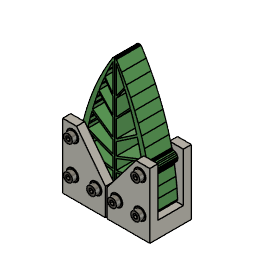
REVIEW_V2_ZeroGap_M3x30 (Autodesk Fusion 360 design; units mm, degrees)
part number: 2026-09-04-15-12-13-781
part number: 2026-09-04-15-12-27-275
part number: 2026-09-04-15-12-29-355
part number: 2026-09-04-15-12-34-345
part number: 2026-09-04-15-12-35-918
Autodesk Fusion 360 part; units mm, degrees
sketch "Single continuous Robotiq-to-UMI adapter envelope" plane through (0, 0, 0) normal (1, 0, 0) x (0, 0, -1) in component "LEFT V2 handed finger"
  line L0 (1, 0) -> (-25.7, 0)
  line L1 (-25.7, 0) -> (-25.7, 40.5)
  line L2 (-25.7, 40.5) -> (-17, 40.5)
  line L3 (-17, 40.5) -> (1, 17)
  line L4 (1, 17) -> (1, 0)
extrude "Extrude1" add sketch "Single continuous Robotiq-to-UMI adapter envelope" along normal mid plane 26 makes body 1 in component "LEFT V2 handed finger"
sketch "Continuous TPU pocket - 0.20 mm clearance per side" plane through (0, 0, 0) normal (0, 0, 1) x (1, 0, 0) in component "LEFT V2 handed finger"
  line L0 (-7.94, 10) -> (7.94, 10)
  line L1 (7.94, 10) -> (7.94, 100)
  line L2 (7.94, 100) -> (-7.94, 100)
  line L3 (-7.94, 100) -> (-7.94, 10)
extrude "Extrude2" cut sketch "Continuous TPU pocket - 0.20 mm clearance per side" along normal mid plane 100 bodies 1 in component "LEFT V2 handed finger"
sketch "Exact Robotiq M5 and indexing interface" plane through (0, 0, 0) normal (0, 1, 0) x (1, 0, 0) in component "LEFT V2 handed finger"
  circle A0 centre (0, -12.36) radius 2.65
  circle A1 centre (-4.5, -12.36) radius 1
  circle A2 centre (4.5, -12.36) radius 1
extrude "Extrude3" cut sketch "Exact Robotiq M5 and indexing interface" along normal blind 4 contours A0 bodies 1 in component "LEFT V2 handed finger"
extrude "Extrude4" cut sketch "Exact Robotiq M5 and indexing interface" along normal blind 2.5 contours A1 | A2 bodies 1 in component "LEFT V2 handed finger"
ref_plane "WorkPlane1" through (0, 4, 0) normal (0, 1, 0) x (0, 0, 1) in component "LEFT V2 handed finger"
sketch "Robotiq M5 SHCS head pocket - 9.2 mm" plane through (0, 4, 0) normal (0, 1, 0) x (1, 0, 0) in component "LEFT V2 handed finger"
  circle A0 centre (0, -12.36) radius 4.6
extrude "Extrude5" cut sketch "Robotiq M5 SHCS head pocket - 9.2 mm" along normal blind 6 bodies 1 in component "LEFT V2 handed finger"
sketch "Three UMI M3 holder clearances - 3.6 mm" plane through (0, 0, 0) normal (1, 0, 0) x (0, 0, -1) in component "LEFT V2 handed finger"
  circle A0 centre (-5, 13) radius 1.8
  circle A1 centre (-19.5, 13) radius 1.8
  circle A2 centre (-19.5, 34) radius 1.8
extrude "Extrude6" cut sketch "Three UMI M3 holder clearances - 3.6 mm" along normal mid plane 30 bodies 1 in component "LEFT V2 handed finger"
ref_plane "WorkPlane2" through (13, 0, 0) normal (1, 0, 0) x (0, 1, 0) in component "LEFT V2 handed finger"
sketch "Three shallow washer seats - 7.5 mm" plane through (13, 0, 0) normal (1, 0, 0) x (0, 0, -1) in component "LEFT V2 handed finger"
  circle A0 centre (-5, 13) radius 3.75
  circle A1 centre (-19.5, 13) radius 3.75
  circle A2 centre (-19.5, 34) radius 3.75
extrude "Extrude7" cut sketch "Three shallow washer seats - 7.5 mm" against normal blind 0.6 bodies 1 in component "LEFT V2 handed finger"
ref_plane "WorkPlane3" through (-13, 0, 0) normal (1, 0, 0) x (0, 1, 0) in component "LEFT V2 handed finger"
sketch "Three enclosed UMI M3 captive-nut pockets - 6.3 mm AF" plane through (-13, 0, 0) normal (1, 0, 0) x (0, 0, -1) in component "LEFT V2 handed finger"
  line L0 (-5, 16.6373) -> (-8.15, 14.8187)
  line L1 (-8.15, 14.8187) -> (-8.15, 11.1813)
  line L2 (-8.15, 11.1813) -> (-5, 9.3627)
  line L3 (-5, 9.3627) -> (-1.85, 11.1813)
  line L4 (-1.85, 11.1813) -> (-1.85, 14.8187)
  line L5 (-1.85, 14.8187) -> (-5, 16.6373)
  line L6 (-19.5, 16.6373) -> (-22.65, 14.8187)
  line L7 (-22.65, 14.8187) -> (-22.65, 11.1813)
  line L8 (-22.65, 11.1813) -> (-19.5, 9.3627)
  line L9 (-19.5, 9.3627) -> (-16.35, 11.1813)
  line L10 (-16.35, 11.1813) -> (-16.35, 14.8187)
  line L11 (-16.35, 14.8187) -> (-19.5, 16.6373)
  line L12 (-19.5, 37.6373) -> (-22.65, 35.8187)
  line L13 (-22.65, 35.8187) -> (-22.65, 32.1813)
  line L14 (-22.65, 32.1813) -> (-19.5, 30.3627)
  line L15 (-19.5, 30.3627) -> (-16.35, 32.1813)
  line L16 (-16.35, 32.1813) -> (-16.35, 35.8187)
  line L17 (-16.35, 35.8187) -> (-19.5, 37.6373)
extrude "Extrude8" cut sketch "Three enclosed UMI M3 captive-nut pockets - 6.3 mm AF" along normal blind 2.5 bodies 1 in component "LEFT V2 handed finger"
sketch "Exact 0.600 UMI exterior at zero-gap datum" plane through (0, 0, 0) normal (1, 0, 0) x (0, 0, -1) in component "LEFT V2 handed finger"
  line L0 (-20.5344, 10) -> (-0.2215, 10.0017)
  line L1 (-0.2215, 10.0017) -> (0.3156, 10.1086)
  line L2 (0.3156, 10.1086) -> (0.8264, 10.3965)
  line L3 (0.8264, 10.3965) -> (1.2181, 10.8329)
  line L4 (1.2181, 10.8329) -> (1.4387, 11.3341)
  line L5 (1.4387, 11.3341) -> (1.5, 11.8)
  line L6 (1.5, 11.8) -> (1.5, 83.4188)
  line L7 (1.5, 83.4188) -> (1.4557, 83.6451)
  line L8 (1.4557, 83.6451) -> (1.3292, 83.838)
  line L9 (1.3292, 83.838) -> (1.1394, 83.969)
  line L10 (1.1394, 83.969) -> (0.9013, 84.0187)
  line L11 (0.9013, 84.0187) -> (0.6165, 83.9476)
  line L12 (0.6165, 83.9476) -> (0.3926, 83.739)
  line L13 (0.3926, 83.739) -> (-2.7977, 78.4418)
  line L14 (-2.7977, 78.4418) -> (-5.7647, 73.0163)
  line L15 (-5.7647, 73.0163) -> (-8.5032, 67.472)
  line L16 (-8.5032, 67.472) -> (-11.0085, 61.8185)
  line L17 (-11.0085, 61.8185) -> (-13.2762, 56.0656)
  line L18 (-13.2762, 56.0656) -> (-15.3023, 50.2232)
  line L19 (-15.3023, 50.2232) -> (-17.0834, 44.3015)
  line L20 (-17.0834, 44.3015) -> (-18.7439, 37.9469)
  line L21 (-18.7439, 37.9469) -> (-19.0202, 37.5295)
  line L22 (-19.0202, 37.5295) -> (-19.4002, 37.2037)
  line L23 (-19.4002, 37.2037) -> (-19.7455, 37.0321)
  line L24 (-19.7455, 37.0321) -> (-20.7817, 36.7124)
  line L25 (-20.7817, 36.7124) -> (-21.4344, 36.293)
  line L26 (-21.4344, 36.293) -> (-22.0298, 35.6125)
  line L27 (-22.0298, 35.6125) -> (-22.3954, 34.7854)
  line L28 (-22.3954, 34.7854) -> (-22.4873, 34.2756)
  line L29 (-22.4873, 34.2756) -> (-22.4902, 33.7575)
  line L30 (-22.4902, 33.7575) -> (-22.4039, 33.2467)
  line L31 (-22.4039, 33.2467) -> (-22.231, 32.7584)
  line L32 (-22.231, 32.7584) -> (-21.737, 32.001)
  line L33 (-21.737, 32.001) -> (-20.7011, 31.0732)
  line L34 (-20.7011, 31.0732) -> (-20.4451, 30.599)
  line L35 (-20.4451, 30.599) -> (-20.3461, 30.1474)
  line L36 (-20.3461, 30.1474) -> (-20.3539, 29.7619)
  line L37 (-20.3539, 29.7619) -> (-21.2594, 23.7815)
  line L38 (-21.2594, 23.7815) -> (-21.9154, 17.8463)
  line L39 (-21.9154, 17.8463) -> (-22.3344, 11.8128)
  line L40 (-22.3344, 11.8128) -> (-22.2082, 11.1378)
  line L41 (-22.2082, 11.1378) -> (-22.0302, 10.7986)
  line L42 (-22.0302, 10.7986) -> (-21.7844, 10.5048)
  line L43 (-21.7844, 10.5048) -> (-21.2084, 10.131)
  line L44 (-21.2084, 10.131) -> (-20.5344, 10)
extrude "Extrude9" add sketch "Exact 0.600 UMI exterior at zero-gap datum" along normal mid plane 15.48 separate body makes body 2 in component "LEFT V2 handed finger"
sketch "Six unchanged UMI-derived through-bays" plane through (0, 0, 0) normal (1, 0, 0) x (0, 0, -1) in component "LEFT V2 handed finger"
  line L0 (-17.748, 16) -> (0.42, 16)
  line L1 (0.42, 16) -> (0.42, 22.564)
  line L2 (0.42, 22.564) -> (-17.43, 25.258)
  line L3 (-17.43, 25.258) -> (-17.766, 22.738)
  line L4 (-17.766, 22.738) -> (-17.91, 21.544)
  line L5 (-17.91, 21.544) -> (-18.192, 19)
  line L6 (-18.192, 19) -> (-18.312, 17.8)
  line L7 (-18.312, 17.8) -> (-18.48, 16)
  line L8 (-18.48, 16) -> (-17.748, 16)
  line L9 (-17.262, 26.446) -> (0.42, 23.782)
  line L10 (0.42, 23.782) -> (0.42, 30.214)
  line L11 (0.42, 30.214) -> (-15.492, 36.46)
  line L12 (-15.492, 36.46) -> (-16.008, 33.88)
  line L13 (-16.008, 33.88) -> (-16.23, 32.692)
  line L14 (-16.23, 32.692) -> (-16.674, 30.154)
  line L15 (-16.674, 30.154) -> (-16.872, 28.966)
  line L16 (-16.872, 28.966) -> (-17.262, 26.446)
  line L17 (-15.24, 37.648) -> (0.42, 31.504)
  line L18 (0.42, 31.504) -> (0.42, 39.364)
  line L19 (0.42, 39.364) -> (-12.63, 48.256)
  line L20 (-12.63, 48.256) -> (-13.398, 45.424)
  line L21 (-13.398, 45.424) -> (-13.71, 44.218)
  line L22 (-13.71, 44.218) -> (-14.376, 41.488)
  line L23 (-14.376, 41.488) -> (-14.658, 40.288)
  line L24 (-14.658, 40.288) -> (-15.24, 37.648)
  line L25 (-12.282, 49.474) -> (0.42, 40.816)
  line L26 (0.42, 40.816) -> (0.42, 51.628)
  line L27 (0.42, 51.628) -> (-8.514, 61.084)
  line L28 (-8.514, 61.084) -> (-9.75, 57.562)
  line L29 (-9.75, 57.562) -> (-10.002, 56.818)
  line L30 (-10.002, 56.818) -> (-11.022, 53.68)
  line L31 (-11.022, 53.68) -> (-11.4, 52.45)
  line L32 (-11.4, 52.45) -> (-12.282, 49.474)
  line L33 (-8.232, 61.84) -> (0.42, 52.678)
  line L34 (0.42, 52.678) -> (0.42, 62.842)
  line L35 (0.42, 62.842) -> (-4.896, 70.222)
  line L36 (-4.896, 70.222) -> (-6.516, 66.31)
  line L37 (-6.516, 66.31) -> (-6.822, 65.548)
  line L38 (-6.822, 65.548) -> (-8.232, 61.84)
  line L39 (-4.566, 70.99) -> (0.42, 64.078)
  line L40 (0.42, 64.078) -> (0.42, 81.52)
  line L41 (0.42, 81.52) -> (-2.34, 75.91)
  line L42 (-2.34, 75.91) -> (-2.706, 75.13)
  line L43 (-2.706, 75.13) -> (-4.566, 70.99)
extrude "Extrude10" cut sketch "Six unchanged UMI-derived through-bays" along normal mid plane 24 bodies 2 in component "LEFT V2 handed finger"
sketch "Three UMI TPU M3 clearances - 4.0 mm" plane through (0, 0, 0) normal (1, 0, 0) x (0, 0, -1) in component "LEFT V2 handed finger"
  circle A0 centre (-5, 13) radius 2
  circle A1 centre (-19.5, 13) radius 2
  circle A2 centre (-19.5, 34) radius 2
extrude "Extrude11" cut sketch "Three UMI TPU M3 clearances - 4.0 mm" along normal mid plane 24 bodies 2 in component "LEFT V2 handed finger"
sketch "Single continuous Robotiq-to-UMI adapter envelope (2)" plane through (0, 0, 0) normal (1, 0, 0) x (0, 0, -1) in component "RIGHT V2 handed finger"
  line L0 (1, 0) -> (-25.7, 0)
  line L1 (-25.7, 0) -> (-25.7, 40.5)
  line L2 (-25.7, 40.5) -> (-17, 40.5)
  line L3 (-17, 40.5) -> (1, 17)
  line L4 (1, 17) -> (1, 0)
extrude "Extrude1'" add sketch "Single continuous Robotiq-to-UMI adapter envelope (2)" along normal mid plane 26 separate body makes body 3 in component "RIGHT V2 handed finger"
sketch "Continuous TPU pocket - 0.20 mm clearance per side (2)" plane through (0, 0, 0) normal (0, 0, 1) x (1, 0, 0) in component "RIGHT V2 handed finger"
  line L0 (-7.94, 10) -> (7.94, 10)
  line L1 (7.94, 10) -> (7.94, 100)
  line L2 (7.94, 100) -> (-7.94, 100)
  line L3 (-7.94, 100) -> (-7.94, 10)
extrude "Extrude2'" cut sketch "Continuous TPU pocket - 0.20 mm clearance per side (2)" along normal mid plane 100 bodies 3 in component "RIGHT V2 handed finger"
sketch "Exact Robotiq M5 and indexing interface (2)" plane through (0, 0, 0) normal (0, 1, 0) x (1, 0, 0) in component "RIGHT V2 handed finger"
  circle A0 centre (0, -12.36) radius 2.65
  circle A1 centre (-4.5, -12.36) radius 1
  circle A2 centre (4.5, -12.36) radius 1
extrude "Extrude3'" cut sketch "Exact Robotiq M5 and indexing interface (2)" along normal blind 4 contours A0 bodies 3 in component "RIGHT V2 handed finger"
extrude "Extrude4'" cut sketch "Exact Robotiq M5 and indexing interface (2)" along normal blind 2.5 contours A1 | A2 bodies 3 in component "RIGHT V2 handed finger"
ref_plane "WorkPlane1" through (0, 4, 0) normal (0, 1, 0) x (0, 0, 1) in component "RIGHT V2 handed finger"
sketch "Robotiq M5 SHCS head pocket - 9.2 mm (2)" plane through (0, 4, 0) normal (0, 1, 0) x (1, 0, 0) in component "RIGHT V2 handed finger"
  circle A0 centre (0, -12.36) radius 4.6
extrude "Extrude5'" cut sketch "Robotiq M5 SHCS head pocket - 9.2 mm (2)" along normal blind 6 bodies 3 in component "RIGHT V2 handed finger"
sketch "Three UMI M3 holder clearances - 3.6 mm (2)" plane through (0, 0, 0) normal (1, 0, 0) x (0, 0, -1) in component "RIGHT V2 handed finger"
  circle A0 centre (-5, 13) radius 1.8
  circle A1 centre (-19.5, 13) radius 1.8
  circle A2 centre (-19.5, 34) radius 1.8
extrude "Extrude6'" cut sketch "Three UMI M3 holder clearances - 3.6 mm (2)" along normal mid plane 30 bodies 3 in component "RIGHT V2 handed finger"
ref_plane "WorkPlane2" through (-13, 0, 0) normal (1, 0, 0) x (0, 1, 0) in component "RIGHT V2 handed finger"
sketch "Three shallow washer seats - 7.5 mm (2)" plane through (-13, 0, 0) normal (1, 0, 0) x (0, 0, -1) in component "RIGHT V2 handed finger"
  circle A0 centre (-5, 13) radius 3.75
  circle A1 centre (-19.5, 13) radius 3.75
  circle A2 centre (-19.5, 34) radius 3.75
extrude "Extrude7'" cut sketch "Three shallow washer seats - 7.5 mm (2)" along normal blind 0.6 bodies 3 in component "RIGHT V2 handed finger"
ref_plane "WorkPlane3" through (13, 0, 0) normal (1, 0, 0) x (0, 1, 0) in component "RIGHT V2 handed finger"
sketch "Three enclosed UMI M3 captive-nut pockets - 6.3 mm AF (2)" plane through (13, 0, 0) normal (1, 0, 0) x (0, 0, -1) in component "RIGHT V2 handed finger"
  line L0 (-5, 16.6373) -> (-8.15, 14.8187)
  line L1 (-8.15, 14.8187) -> (-8.15, 11.1813)
  line L2 (-8.15, 11.1813) -> (-5, 9.3627)
  line L3 (-5, 9.3627) -> (-1.85, 11.1813)
  line L4 (-1.85, 11.1813) -> (-1.85, 14.8187)
  line L5 (-1.85, 14.8187) -> (-5, 16.6373)
  line L6 (-19.5, 16.6373) -> (-22.65, 14.8187)
  line L7 (-22.65, 14.8187) -> (-22.65, 11.1813)
  line L8 (-22.65, 11.1813) -> (-19.5, 9.3627)
  line L9 (-19.5, 9.3627) -> (-16.35, 11.1813)
  line L10 (-16.35, 11.1813) -> (-16.35, 14.8187)
  line L11 (-16.35, 14.8187) -> (-19.5, 16.6373)
  line L12 (-19.5, 37.6373) -> (-22.65, 35.8187)
  line L13 (-22.65, 35.8187) -> (-22.65, 32.1813)
  line L14 (-22.65, 32.1813) -> (-19.5, 30.3627)
  line L15 (-19.5, 30.3627) -> (-16.35, 32.1813)
  line L16 (-16.35, 32.1813) -> (-16.35, 35.8187)
  line L17 (-16.35, 35.8187) -> (-19.5, 37.6373)
extrude "Extrude8'" cut sketch "Three enclosed UMI M3 captive-nut pockets - 6.3 mm AF (2)" against normal blind 2.5 bodies 3 in component "RIGHT V2 handed finger"
sketch "Exact 0.600 UMI exterior at zero-gap datum (2)" plane through (0, 0, 0) normal (1, 0, 0) x (0, 0, -1) in component "RIGHT V2 handed finger"
  line L0 (-20.5344, 10) -> (-0.2215, 10.0017)
  line L1 (-0.2215, 10.0017) -> (0.3156, 10.1086)
  line L2 (0.3156, 10.1086) -> (0.8264, 10.3965)
  line L3 (0.8264, 10.3965) -> (1.2181, 10.8329)
  line L4 (1.2181, 10.8329) -> (1.4387, 11.3341)
  line L5 (1.4387, 11.3341) -> (1.5, 11.8)
  line L6 (1.5, 11.8) -> (1.5, 83.4188)
  line L7 (1.5, 83.4188) -> (1.4557, 83.6451)
  line L8 (1.4557, 83.6451) -> (1.3292, 83.838)
  line L9 (1.3292, 83.838) -> (1.1394, 83.969)
  line L10 (1.1394, 83.969) -> (0.9013, 84.0187)
  line L11 (0.9013, 84.0187) -> (0.6165, 83.9476)
  line L12 (0.6165, 83.9476) -> (0.3926, 83.739)
  line L13 (0.3926, 83.739) -> (-2.7977, 78.4418)
  line L14 (-2.7977, 78.4418) -> (-5.7647, 73.0163)
  line L15 (-5.7647, 73.0163) -> (-8.5032, 67.472)
  line L16 (-8.5032, 67.472) -> (-11.0085, 61.8185)
  line L17 (-11.0085, 61.8185) -> (-13.2762, 56.0656)
  line L18 (-13.2762, 56.0656) -> (-15.3023, 50.2232)
  line L19 (-15.3023, 50.2232) -> (-17.0834, 44.3015)
  line L20 (-17.0834, 44.3015) -> (-18.7439, 37.9469)
  line L21 (-18.7439, 37.9469) -> (-19.0202, 37.5295)
  line L22 (-19.0202, 37.5295) -> (-19.4002, 37.2037)
  line L23 (-19.4002, 37.2037) -> (-19.7455, 37.0321)
  line L24 (-19.7455, 37.0321) -> (-20.7817, 36.7124)
  line L25 (-20.7817, 36.7124) -> (-21.4344, 36.293)
  line L26 (-21.4344, 36.293) -> (-22.0298, 35.6125)
  line L27 (-22.0298, 35.6125) -> (-22.3954, 34.7854)
  line L28 (-22.3954, 34.7854) -> (-22.4873, 34.2756)
  line L29 (-22.4873, 34.2756) -> (-22.4902, 33.7575)
  line L30 (-22.4902, 33.7575) -> (-22.4039, 33.2467)
  line L31 (-22.4039, 33.2467) -> (-22.231, 32.7584)
  line L32 (-22.231, 32.7584) -> (-21.737, 32.001)
  line L33 (-21.737, 32.001) -> (-20.7011, 31.0732)
  line L34 (-20.7011, 31.0732) -> (-20.4451, 30.599)
  line L35 (-20.4451, 30.599) -> (-20.3461, 30.1474)
  line L36 (-20.3461, 30.1474) -> (-20.3539, 29.7619)
  line L37 (-20.3539, 29.7619) -> (-21.2594, 23.7815)
  line L38 (-21.2594, 23.7815) -> (-21.9154, 17.8463)
  line L39 (-21.9154, 17.8463) -> (-22.3344, 11.8128)
  line L40 (-22.3344, 11.8128) -> (-22.2082, 11.1378)
  line L41 (-22.2082, 11.1378) -> (-22.0302, 10.7986)
  line L42 (-22.0302, 10.7986) -> (-21.7844, 10.5048)
  line L43 (-21.7844, 10.5048) -> (-21.2084, 10.131)
  line L44 (-21.2084, 10.131) -> (-20.5344, 10)
extrude "Extrude9'" add sketch "Exact 0.600 UMI exterior at zero-gap datum (2)" along normal mid plane 15.48 separate body makes body 4 in component "RIGHT V2 handed finger"
sketch "Six unchanged UMI-derived through-bays (2)" plane through (0, 0, 0) normal (1, 0, 0) x (0, 0, -1) in component "RIGHT V2 handed finger"
  line L0 (-17.748, 16) -> (0.42, 16)
  line L1 (0.42, 16) -> (0.42, 22.564)
  line L2 (0.42, 22.564) -> (-17.43, 25.258)
  line L3 (-17.43, 25.258) -> (-17.766, 22.738)
  line L4 (-17.766, 22.738) -> (-17.91, 21.544)
  line L5 (-17.91, 21.544) -> (-18.192, 19)
  line L6 (-18.192, 19) -> (-18.312, 17.8)
  line L7 (-18.312, 17.8) -> (-18.48, 16)
  line L8 (-18.48, 16) -> (-17.748, 16)
  line L9 (-17.262, 26.446) -> (0.42, 23.782)
  line L10 (0.42, 23.782) -> (0.42, 30.214)
  line L11 (0.42, 30.214) -> (-15.492, 36.46)
  line L12 (-15.492, 36.46) -> (-16.008, 33.88)
  line L13 (-16.008, 33.88) -> (-16.23, 32.692)
  line L14 (-16.23, 32.692) -> (-16.674, 30.154)
  line L15 (-16.674, 30.154) -> (-16.872, 28.966)
  line L16 (-16.872, 28.966) -> (-17.262, 26.446)
  line L17 (-15.24, 37.648) -> (0.42, 31.504)
  line L18 (0.42, 31.504) -> (0.42, 39.364)
  line L19 (0.42, 39.364) -> (-12.63, 48.256)
  line L20 (-12.63, 48.256) -> (-13.398, 45.424)
  line L21 (-13.398, 45.424) -> (-13.71, 44.218)
  line L22 (-13.71, 44.218) -> (-14.376, 41.488)
  line L23 (-14.376, 41.488) -> (-14.658, 40.288)
  line L24 (-14.658, 40.288) -> (-15.24, 37.648)
  line L25 (-12.282, 49.474) -> (0.42, 40.816)
  line L26 (0.42, 40.816) -> (0.42, 51.628)
  line L27 (0.42, 51.628) -> (-8.514, 61.084)
  line L28 (-8.514, 61.084) -> (-9.75, 57.562)
  line L29 (-9.75, 57.562) -> (-10.002, 56.818)
  line L30 (-10.002, 56.818) -> (-11.022, 53.68)
  line L31 (-11.022, 53.68) -> (-11.4, 52.45)
  line L32 (-11.4, 52.45) -> (-12.282, 49.474)
  line L33 (-8.232, 61.84) -> (0.42, 52.678)
  line L34 (0.42, 52.678) -> (0.42, 62.842)
  line L35 (0.42, 62.842) -> (-4.896, 70.222)
  line L36 (-4.896, 70.222) -> (-6.516, 66.31)
  line L37 (-6.516, 66.31) -> (-6.822, 65.548)
  line L38 (-6.822, 65.548) -> (-8.232, 61.84)
  line L39 (-4.566, 70.99) -> (0.42, 64.078)
  line L40 (0.42, 64.078) -> (0.42, 81.52)
  line L41 (0.42, 81.52) -> (-2.34, 75.91)
  line L42 (-2.34, 75.91) -> (-2.706, 75.13)
  line L43 (-2.706, 75.13) -> (-4.566, 70.99)
extrude "Extrude10'" cut sketch "Six unchanged UMI-derived through-bays (2)" along normal mid plane 24 bodies 4 in component "RIGHT V2 handed finger"
sketch "Three UMI TPU M3 clearances - 4.0 mm (2)" plane through (0, 0, 0) normal (1, 0, 0) x (0, 0, -1) in component "RIGHT V2 handed finger"
  circle A0 centre (-5, 13) radius 2
  circle A1 centre (-19.5, 13) radius 2
  circle A2 centre (-19.5, 34) radius 2
extrude "Extrude11'" cut sketch "Three UMI TPU M3 clearances - 4.0 mm (2)" along normal mid plane 24 bodies 4 in component "RIGHT V2 handed finger"
ref_plane "WorkPlane1" through (12.9, 0, 0) normal (1, 0, 0) x (0, 1, 0) in component "REFERENCE hardware LEFT - M3x30, nominal 7x0.5 washers"
sketch "Nominal M3 socket heads - 5.5 x 3 mm" plane through (12.9, 0, 0) normal (1, 0, 0) x (0, 0, -1) in component "REFERENCE hardware LEFT - M3x30, nominal 7x0.5 washers"
  circle A0 centre (-5, 13) radius 2.75
  circle A1 centre (-19.5, 13) radius 2.75
  circle A2 centre (-19.5, 34) radius 2.75
extrude "Extrude1''" add sketch "Nominal M3 socket heads - 5.5 x 3 mm" along normal blind 3 separate body makes body 5 at (14.9, 12.8629, 2.2534) makes body 6 at (14.9, 12.8629, 16.7534) makes body 7 at (14.9, 33.8629, 16.7534) in component "REFERENCE hardware LEFT - M3x30, nominal 7x0.5 washers"
ref_plane "WorkPlane2" through (12.9, 0, 0) normal (1, 0, 0) x (0, 1, 0) in component "REFERENCE hardware LEFT - M3x30, nominal 7x0.5 washers"
sketch "Full 30 mm screw shanks" plane through (12.9, 0, 0) normal (1, 0, 0) x (0, 0, -1) in component "REFERENCE hardware LEFT - M3x30, nominal 7x0.5 washers"
  circle A0 centre (-5, 13) radius 1.5
  circle A1 centre (-19.5, 13) radius 1.5
  circle A2 centre (-19.5, 34) radius 1.5
extrude "Extrude2''" add sketch "Full 30 mm screw shanks" against normal blind 30 bodies 5 6 7 in component "REFERENCE hardware LEFT - M3x30, nominal 7x0.5 washers"
ref_plane "WorkPlane3" through (15.9, 0, 0) normal (1, 0, 0) x (0, 1, 0) in component "REFERENCE hardware LEFT - M3x30, nominal 7x0.5 washers"
sketch "2.5 mm hex keys - visual reference" plane through (15.9, 0, 0) normal (1, 0, 0) x (0, 0, -1) in component "REFERENCE hardware LEFT - M3x30, nominal 7x0.5 washers"
  line L0 (-5, 14.4434) -> (-6.25, 13.7217)
  line L1 (-6.25, 13.7217) -> (-6.25, 12.2783)
  line L2 (-6.25, 12.2783) -> (-5, 11.5566)
  line L3 (-5, 11.5566) -> (-3.75, 12.2783)
  line L4 (-3.75, 12.2783) -> (-3.75, 13.7217)
  line L5 (-3.75, 13.7217) -> (-5, 14.4434)
  line L6 (-19.5, 14.4434) -> (-20.75, 13.7217)
  line L7 (-20.75, 13.7217) -> (-20.75, 12.2783)
  line L8 (-20.75, 12.2783) -> (-19.5, 11.5566)
  line L9 (-19.5, 11.5566) -> (-18.25, 12.2783)
  line L10 (-18.25, 12.2783) -> (-18.25, 13.7217)
  line L11 (-18.25, 13.7217) -> (-19.5, 14.4434)
  line L12 (-19.5, 35.4434) -> (-20.75, 34.7217)
  line L13 (-20.75, 34.7217) -> (-20.75, 33.2783)
  line L14 (-20.75, 33.2783) -> (-19.5, 32.5566)
  line L15 (-19.5, 32.5566) -> (-18.25, 33.2783)
  line L16 (-18.25, 33.2783) -> (-18.25, 34.7217)
  line L17 (-18.25, 34.7217) -> (-19.5, 35.4434)
extrude "Extrude3''" cut sketch "2.5 mm hex keys - visual reference" against normal blind 1.5 bodies 5 6 7 in component "REFERENCE hardware LEFT - M3x30, nominal 7x0.5 washers"
ref_plane "WorkPlane4" through (12.4, 0, 0) normal (1, 0, 0) x (0, 1, 0) in component "REFERENCE hardware LEFT - M3x30, nominal 7x0.5 washers"
sketch "Provisional M3 washers - OD7 ID3.2 t0.5" plane through (12.4, 0, 0) normal (1, 0, 0) x (0, 0, -1) in component "REFERENCE hardware LEFT - M3x30, nominal 7x0.5 washers"
  circle A0 centre (-5, 13) radius 3.5
  circle A1 centre (-5, 13) radius 1.6
  circle A2 centre (-19.5, 13) radius 3.5
  circle A3 centre (-19.5, 13) radius 1.6
  circle A4 centre (-19.5, 34) radius 3.5
  circle A5 centre (-19.5, 34) radius 1.6
extrude "Extrude4''" add sketch "Provisional M3 washers - OD7 ID3.2 t0.5" along normal blind 0.5 separate body makes body 8 at (12.4, 12.8261, 2.1464) makes body 9 at (12.4, 12.7466, 16.6523) makes body 10 at (12.4, 33.7466, 16.6523) in component "REFERENCE hardware LEFT - M3x30, nominal 7x0.5 washers"
ref_plane "WorkPlane5" through (-10.5, 0, 0) normal (1, 0, 0) x (0, 1, 0) in component "REFERENCE hardware LEFT - M3x30, nominal 7x0.5 washers"
sketch "Nominal M3 nuts - AF5.5 x 2.4 mm" plane through (-10.5, 0, 0) normal (1, 0, 0) x (0, 0, -1) in component "REFERENCE hardware LEFT - M3x30, nominal 7x0.5 washers"
  line L0 (-5, 16.1754) -> (-7.75, 14.5877)
  line L1 (-7.75, 14.5877) -> (-7.75, 11.4123)
  line L2 (-7.75, 11.4123) -> (-5, 9.8246)
  line L3 (-5, 9.8246) -> (-2.25, 11.4123)
  line L4 (-2.25, 11.4123) -> (-2.25, 14.5877)
  line L5 (-2.25, 14.5877) -> (-5, 16.1754)
  circle A0 centre (-5, 13) radius 1.6
  line L6 (-19.5, 16.1754) -> (-22.25, 14.5877)
  line L7 (-22.25, 14.5877) -> (-22.25, 11.4123)
  line L8 (-22.25, 11.4123) -> (-19.5, 9.8246)
  line L9 (-19.5, 9.8246) -> (-16.75, 11.4123)
  line L10 (-16.75, 11.4123) -> (-16.75, 14.5877)
  line L11 (-16.75, 14.5877) -> (-19.5, 16.1754)
  circle A1 centre (-19.5, 13) radius 1.6
  line L12 (-19.5, 37.1754) -> (-22.25, 35.5877)
  line L13 (-22.25, 35.5877) -> (-22.25, 32.4123)
  line L14 (-22.25, 32.4123) -> (-19.5, 30.8246)
  line L15 (-19.5, 30.8246) -> (-16.75, 32.4123)
  line L16 (-16.75, 32.4123) -> (-16.75, 35.5877)
  line L17 (-16.75, 35.5877) -> (-19.5, 37.1754)
  circle A2 centre (-19.5, 34) radius 1.6
extrude "Extrude5''" add sketch "Nominal M3 nuts - AF5.5 x 2.4 mm" against normal blind 2.4 separate body makes body 11 at (-12.1, 12.9202, 3.402) makes body 12 at (-12.1, 12.9202, 17.902) makes body 13 at (-12.1, 34.7652, 20.9052) in component "REFERENCE hardware LEFT - M3x30, nominal 7x0.5 washers"
ref_plane "WorkPlane1" through (-12.9, 0, 0) normal (1, 0, 0) x (0, 1, 0) in component "REFERENCE hardware RIGHT - M3x30, nominal 7x0.5 washers"
sketch "Nominal M3 socket heads - 5.5 x 3 mm (2)" plane through (-12.9, 0, 0) normal (1, 0, 0) x (0, 0, -1) in component "REFERENCE hardware RIGHT - M3x30, nominal 7x0.5 washers"
  circle A0 centre (-5, 13) radius 2.75
  circle A1 centre (-19.5, 13) radius 2.75
  circle A2 centre (-19.5, 34) radius 2.75
extrude "Extrude1'''" add sketch "Nominal M3 socket heads - 5.5 x 3 mm (2)" against normal blind 3 separate body makes body 14 at (-14.9, 12.8629, 2.2534) makes body 15 at (-14.9, 12.8629, 16.7534) makes body 16 at (-14.9, 33.8629, 16.7534) in component "REFERENCE hardware RIGHT - M3x30, nominal 7x0.5 washers"
ref_plane "WorkPlane2" through (-12.9, 0, 0) normal (1, 0, 0) x (0, 1, 0) in component "REFERENCE hardware RIGHT - M3x30, nominal 7x0.5 washers"
sketch "Full 30 mm screw shanks (2)" plane through (-12.9, 0, 0) normal (1, 0, 0) x (0, 0, -1) in component "REFERENCE hardware RIGHT - M3x30, nominal 7x0.5 washers"
  circle A0 centre (-5, 13) radius 1.5
  circle A1 centre (-19.5, 13) radius 1.5
  circle A2 centre (-19.5, 34) radius 1.5
extrude "Extrude2'''" add sketch "Full 30 mm screw shanks (2)" along normal blind 30 bodies 14 15 16 in component "REFERENCE hardware RIGHT - M3x30, nominal 7x0.5 washers"
ref_plane "WorkPlane3" through (-15.9, 0, 0) normal (1, 0, 0) x (0, 1, 0) in component "REFERENCE hardware RIGHT - M3x30, nominal 7x0.5 washers"
sketch "2.5 mm hex keys - visual reference (2)" plane through (-15.9, 0, 0) normal (1, 0, 0) x (0, 0, -1) in component "REFERENCE hardware RIGHT - M3x30, nominal 7x0.5 washers"
  line L0 (-5, 14.4434) -> (-6.25, 13.7217)
  line L1 (-6.25, 13.7217) -> (-6.25, 12.2783)
  line L2 (-6.25, 12.2783) -> (-5, 11.5566)
  line L3 (-5, 11.5566) -> (-3.75, 12.2783)
  line L4 (-3.75, 12.2783) -> (-3.75, 13.7217)
  line L5 (-3.75, 13.7217) -> (-5, 14.4434)
  line L6 (-19.5, 14.4434) -> (-20.75, 13.7217)
  line L7 (-20.75, 13.7217) -> (-20.75, 12.2783)
  line L8 (-20.75, 12.2783) -> (-19.5, 11.5566)
  line L9 (-19.5, 11.5566) -> (-18.25, 12.2783)
  line L10 (-18.25, 12.2783) -> (-18.25, 13.7217)
  line L11 (-18.25, 13.7217) -> (-19.5, 14.4434)
  line L12 (-19.5, 35.4434) -> (-20.75, 34.7217)
  line L13 (-20.75, 34.7217) -> (-20.75, 33.2783)
  line L14 (-20.75, 33.2783) -> (-19.5, 32.5566)
  line L15 (-19.5, 32.5566) -> (-18.25, 33.2783)
  line L16 (-18.25, 33.2783) -> (-18.25, 34.7217)
  line L17 (-18.25, 34.7217) -> (-19.5, 35.4434)
extrude "Extrude3'''" cut sketch "2.5 mm hex keys - visual reference (2)" along normal blind 1.5 bodies 14 15 16 in component "REFERENCE hardware RIGHT - M3x30, nominal 7x0.5 washers"
ref_plane "WorkPlane4" through (-12.4, 0, 0) normal (1, 0, 0) x (0, 1, 0) in component "REFERENCE hardware RIGHT - M3x30, nominal 7x0.5 washers"
sketch "Provisional M3 washers - OD7 ID3.2 t0.5 (2)" plane through (-12.4, 0, 0) normal (1, 0, 0) x (0, 0, -1) in component "REFERENCE hardware RIGHT - M3x30, nominal 7x0.5 washers"
  circle A0 centre (-5, 13) radius 3.5
  circle A1 centre (-5, 13) radius 1.6
  circle A2 centre (-19.5, 13) radius 3.5
  circle A3 centre (-19.5, 13) radius 1.6
  circle A4 centre (-19.5, 34) radius 3.5
  circle A5 centre (-19.5, 34) radius 1.6
extrude "Extrude4'''" add sketch "Provisional M3 washers - OD7 ID3.2 t0.5 (2)" against normal blind 0.5 separate body makes body 17 at (-12.4, 12.8261, 2.1464) makes body 18 at (-12.4, 12.7466, 16.6523) makes body 19 at (-12.4, 33.7466, 16.6523) in component "REFERENCE hardware RIGHT - M3x30, nominal 7x0.5 washers"
ref_plane "WorkPlane5" through (10.5, 0, 0) normal (1, 0, 0) x (0, 1, 0) in component "REFERENCE hardware RIGHT - M3x30, nominal 7x0.5 washers"
sketch "Nominal M3 nuts - AF5.5 x 2.4 mm (2)" plane through (10.5, 0, 0) normal (1, 0, 0) x (0, 0, -1) in component "REFERENCE hardware RIGHT - M3x30, nominal 7x0.5 washers"
  line L0 (-5, 16.1754) -> (-7.75, 14.5877)
  line L1 (-7.75, 14.5877) -> (-7.75, 11.4123)
  line L2 (-7.75, 11.4123) -> (-5, 9.8246)
  line L3 (-5, 9.8246) -> (-2.25, 11.4123)
  line L4 (-2.25, 11.4123) -> (-2.25, 14.5877)
  line L5 (-2.25, 14.5877) -> (-5, 16.1754)
  circle A0 centre (-5, 13) radius 1.6
  line L6 (-19.5, 16.1754) -> (-22.25, 14.5877)
  line L7 (-22.25, 14.5877) -> (-22.25, 11.4123)
  line L8 (-22.25, 11.4123) -> (-19.5, 9.8246)
  line L9 (-19.5, 9.8246) -> (-16.75, 11.4123)
  line L10 (-16.75, 11.4123) -> (-16.75, 14.5877)
  line L11 (-16.75, 14.5877) -> (-19.5, 16.1754)
  circle A1 centre (-19.5, 13) radius 1.6
  line L12 (-19.5, 37.1754) -> (-22.25, 35.5877)
  line L13 (-22.25, 35.5877) -> (-22.25, 32.4123)
  line L14 (-22.25, 32.4123) -> (-19.5, 30.8246)
  line L15 (-19.5, 30.8246) -> (-16.75, 32.4123)
  line L16 (-16.75, 32.4123) -> (-16.75, 35.5877)
  line L17 (-16.75, 35.5877) -> (-19.5, 37.1754)
  circle A2 centre (-19.5, 34) radius 1.6
extrude "Extrude5'''" add sketch "Nominal M3 nuts - AF5.5 x 2.4 mm (2)" along normal blind 2.4 separate body makes body 20 at (12.1, 12.9202, 3.402) makes body 21 at (12.1, 12.9202, 17.902) makes body 22 at (12.1, 34.7652, 20.9052) in component "REFERENCE hardware RIGHT - M3x30, nominal 7x0.5 washers"
component "LEFT V2 handed finger" placed x (0, 0, 1) y (0, 1, 0) z (-1, 0, 0) at (-1.5, 124.82, 0)
component "RIGHT V2 handed finger" placed x (0, 0, -1) y (0, 1, 0) z (1, 0, 0) at (1.5, 124.82, 0)
component "REFERENCE hardware LEFT - M3x30, nominal 7x0.5 washers" placed x (1, 0, 0) y (0, 1, 0) z (0, 0, 1) at (0, 0, 0) in component "LEFT V2 handed finger"
component "REFERENCE hardware RIGHT - M3x30, nominal 7x0.5 washers" placed x (1, 0, 0) y (0, 1, 0) z (0, 0, 1) at (0, 0, 0) in component "RIGHT V2 handed finger"
equation "adapterOverallWidth = 26 mm" comment "V2 thicker PETG cheeks"
equation "adapterSlotWidth = 15.88 mm" comment "15.48 mm TPU plus 0.20 mm clearance per side"
equation "tpuFingerThickness = 15.48 mm" comment "Exact 0.600 scale of the UMI 25.8 mm thickness"
equation "adapterM3Clearance = 3.6 mm" comment "UMI holder M3 clearance"
equation "tpuM3Clearance = 4.0 mm" comment "UMI soft-finger M3 clearance"
equation "closedClearancePerSide = 0 mm" comment "Bare TPU rails meet at mechanical closure"
equation "m5ShoulderDepth = 4 mm" comment "Unchanged OEM fingertip shoulder"
equation "m5HeadToolPocketDepth = 6 mm" comment "Reduced from 10 mm for the measured 4.9 mm M5 head"
equation "adapterRootDepth = 10 mm" comment "Unchanged 4 mm shoulder plus 6 mm M5 head pocket"
equation "tpuRootShift = -4 mm" comment "Move TPU base from Y=14 mm to the Y=10 mm PETG split"
equation "adapterDistalExtent = 40.5 mm" comment "Trimmed inward from 42.9 mm at the user's marked PETG edge"
equation "washerSeatDiameter = 7.5 mm" comment "Provisional 7 mm washer plus radial clearance"
equation "washerSeatDepth = 0.6 mm" comment "Shallow seat for provisional 0.5 mm washer"
equation "washerThickness = 0.5 mm" comment "VIGRUE kit dimension not yet measured"
equation "jointScrewLength = 30 mm" comment "Use full-length screws without cutting"
equation "petgClosingClearancePerSide = 0.5 mm" comment "Rigid holders clear each other at TPU contact"
equation "d17 = adapterOverallWidth"
equation "d33 = -( washerSeatDepth )"
equation "d45 = adapterOverallWidth"
equation "d61 = washerSeatDepth"
equation "d65 = -( 2.5 mm )"
equation "d79 = -( 30.0 mm )"
equation "d83 = -( 1.5 mm )"
equation "d91 = -( 2.4 mm )"
equation "d95 = -( 3.0 mm )"
equation "d107 = -( 0.5 mm )"
named bodies: "PETG Adapter LEFT", "TPU 95A Finger LEFT", "PETG Adapter RIGHT", "TPU 95A Finger RIGHT", "M3x30 screw 1 - nominal unthreaded envelope", "M3x30 screw 2 - nominal unthreaded envelope", "M3x30 screw 3 - nominal unthreaded envelope", "M3 washer 1 - PROVISIONAL 7 x 0.5 mm", "M3 washer 2 - PROVISIONAL 7 x 0.5 mm", "M3 washer 3 - PROVISIONAL 7 x 0.5 mm", "M3 nut 1 - nominal thread-free reference", "M3 nut 2 - nominal thread-free reference", "M3 nut 3 - nominal thread-free reference"
